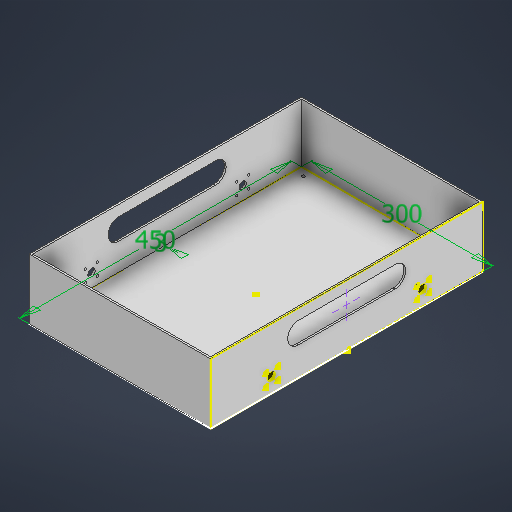
# Autodesk Inventor part: AMR_Base_Box_V2
Saved by Autodesk Inventor 2026.2 (Build 302298010, 298A)
## iProperties
Created: 2026-03-25
Part Number: AMR_Base_Box_V2
Material: Generic
Document SubType Name: Modeling
Designer: Srishanth Dhondy
Density: 1 g/cm^3
Appearance: Default
Author: Srishanth Dhondy
Autodesk Inventor part; units mm, degrees
ref_plane "YZ Plane" through (0, 0, 0) normal (1, 0, 0) x (0, 1, 0)
ref_plane "XZ Plane" through (0, 0, 0) normal (0, 1, 0) x (-1, 0, 0)
ref_plane "XY Plane" through (0, 0, 0) normal (0, 0, 1) x (1, 0, 0)
sketch "Sketch1" plane through (0, 0, 0) normal (0, 1, 0) x (-1, 0, 0)
  line L0 (-150, 225) -> (150, 225)
  line L1 (150, 225) -> (150, -225)
  line L2 (150, -225) -> (-150, -225)
  line L3 (-150, -225) -> (-150, 225)
  line L4 (-150, 225) -> (150, -225) construction
  line L5 (150, 225) -> (-150, -225) construction
  line L6 (147, -222) -> (147, 222)
  line L7 (147, 222) -> (-147, 222)
  line L8 (-147, 222) -> (-147, -222)
  line L9 (-147, -222) -> (147, -222)
  point P0 (0, 0)
  dimension "d0" = 300
  dimension "d1" = 450
  dimension "d4" = 3
  constraints: 20 end point, 4 parallel, 2 midpoint, 2 perpendicular, 1 horizontal, 3 other
  measures "d0" distance of L1.end L2.end
  measures "d1" distance of L0.end L1.end
  measures "d4" distance between parallel lines of L1 L6
extrude "Extrusion1" add sketch "Sketch1" along normal blind 3 contours L0 L1 L2 L3 | L9 L8 L7 L6
extrude "Extrusion2" add sketch "Sketch1" along normal blind 100
sketch "Sketch2" plane through (150, 0, 225) normal (1, 0, 0) x (0, 0, -1)
  line L0 (0, 0) -> (450, 0) projected
  line L1 (450, 0) -> (450, 100) projected
  line L2 (0, 100) -> (450, 100) projected
  line L3 (0, 0) -> (0, 100) projected
  line L4 (0, 25) -> (450, 25)
  circle A0 centre (100, 25) radius 14
  circle A1 centre (350, 25) radius 14
  line L5 (100, 25) -> (109.8995, 34.8995) construction
  line L6 (100, 25) -> (114, 25) construction
  line L7 (225, 100) -> (225, 0) construction
  circle A2 centre (100, 25) radius 6
  circle A3 centre (350, 25) radius 6
  point P0 (90.1005, 34.8995)
  point P1 (90.1005, 15.1005)
  point P2 (109.8995, 15.1005)
  point P3 (340.1005, 34.8995)
  point P4 (359.8995, 34.8995)
  point P5 (359.8995, 15.1005)
  point P6 (340.1005, 15.1005)
  dimension "d7" = 28
  dimension "d8" = 28
  dimension "d9" = 45
  dimension "d12" = 360
  dimension "d14" = 12
  dimension "d15" = 12
  constraints: 13 coincident, 8 end point, 4 point on line, 4 symmetric about line, 3 centre point, 2 perpendicular, 1 equal length, 1 horizontal, 1 midpoint, 8 other
  measures "d8" diameter of A1
  measures "d9" angle of L6 L5
  measures "d14" diameter of A2
  measures "d15" diameter of A3
hole "Hole1" at (150, 25, 125) at (150, 25, -125) direction (-1, 0, 0) diameter 12 end through all
hole "Hole2" at (150, 34.8995, 134.8995) at (150, 15.1005, 115.1005) at (150, 15.1005, 134.8995) at (150, 34.8995, 115.1005) at (150, 34.8995, -115.1005) at (150, 15.1005, -115.1005) at (150, 15.1005, -134.8995) at (150, 34.8995, -134.8995) direction (-1, 0, 0) diameter 3.5 end through all
sketch "Sketch3" plane through (0, 3, 0) normal (0, 1, 0) x (1, 0, 0)
  line L0 (-147, 222) -> (-147, -222) projected
  line L1 (-147, -222) -> (147, -222) projected
  line L2 (147, -222) -> (147, 222) projected
  line L3 (147, 222) -> (-147, 222) projected
  point P0 (0, 0)
sketch "Sketch4" plane through (0, 3, 0) normal (0, 1, 0) x (1, 0, 0)
  line L0 (-147, 222) -> (-147, -222) projected
  line L1 (147, -222) -> (147, 222) projected
  line L2 (150, 225) -> (-150, 225) projected
  line L3 (0, 225) -> (0, -313.1103)
  line L4 (-147, 0) -> (147, 0)
  point P0 (0, 0)
  point P1 (-202.9851, -76.8809)
  point P2 (132, 256.112)
  point P3 (-124.075, 248.076)
  point P4 (-124.075, -228.643)
  point P5 (147.6668, -220.1737)
  point P6 (132, 210)
  point P7 (-132, 210)
  point P8 (132, -210)
  point P9 (-132, -210)
  dimension "d30" = 132
  dimension "d31" = 210
  constraints: 4 end point, 3 midpoint, 3 symmetric about line, 1 vertical
  measures "d30" distance from line of point (132, 256.112) L3
  measures "d31" distance from line of point (132, 210) L4
hole "Hole3" at (132, 3, -210) at (-132, 3, -210) at (-132, 3, 210) at (132, 3, 210) direction (0, -1, 0) diameter 5 end through all
sketch "Sketch5" plane through (150, 0, 225) normal (1, 0, 0) x (0, 0, -1)
  circle A0 centre (359.8995, 34.8995) radius 1.75 projected
  circle A1 centre (359.8995, 15.1005) radius 1.75 projected
  circle A2 centre (340.1005, 15.1005) radius 1.75 projected
  circle A3 centre (340.1005, 34.8995) radius 1.75 projected
  circle A4 centre (109.8995, 34.8995) radius 1.75 projected
  circle A5 centre (90.1005, 15.1005) radius 1.75 projected
  circle A6 centre (109.8995, 15.1005) radius 1.75 projected
  circle A7 centre (90.1005, 34.8995) radius 1.75 projected
  circle A8 centre (350, 25) radius 6 projected
  circle A9 centre (100, 25) radius 6 projected
  line L0 (0, 0) -> (450, 0) projected
  line L1 (450, 0) -> (450, 100) projected
  line L2 (0, 100) -> (450, 100) projected
  line L3 (0, 0) -> (0, 100) projected
  point P0 (225, 0)
  point P1 (225, 65)
  point P2 (225, 65)
  constraints: 1 coincident
sketch "Sketch6" plane through (150, 0, 225) normal (1, 0, 0) x (0, 0, -1)
  circle A0 centre (359.8995, 34.8995) radius 1.75 projected
  circle A1 centre (359.8995, 15.1005) radius 1.75 projected
  circle A2 centre (340.1005, 15.1005) radius 1.75 projected
  circle A3 centre (340.1005, 34.8995) radius 1.75 projected
  circle A4 centre (109.8995, 34.8995) radius 1.75 projected
  circle A5 centre (90.1005, 15.1005) radius 1.75 projected
  circle A6 centre (109.8995, 15.1005) radius 1.75 projected
  circle A7 centre (90.1005, 34.8995) radius 1.75 projected
  circle A8 centre (350, 25) radius 6 projected
  circle A9 centre (100, 25) radius 6 projected
  line L0 (0, 0) -> (450, 0) projected
  line L1 (450, 0) -> (450, 100) projected
  line L2 (0, 100) -> (450, 100) projected
  line L3 (0, 0) -> (0, 100) projected
  point P0 (225, 0)
sketch "Sketch7" plane through (150, 0, 225) normal (1, 0, 0) x (0, 0, -1)
  line L0 (145, 65.0001) -> (305, 65.0001) construction
  line L1 (145, 47.5001) -> (305, 47.5001)
  line L2 (305, 82.5001) -> (145, 82.5001)
  arc A0 (145, 82.5001) -> (145, 47.5001) centre (145, 65.0001) ccw
  arc A1 (305, 47.5001) -> (305, 82.5001) centre (305, 65.0001) ccw
  point P0 (225, 0)
  point P1 (225, 65.0001)
  dimension "d42" = 80
  dimension "d43" = 35
  constraints: 8 end point, 4 point on circle, 4 tangent, 2 centre point, 1 horizontal, 1 midpoint, 1 parallel
  measures "d42" distance of point (225, 65) L0.end
  measures "d43" diameter of A1
extrude "Extrusion3" cut sketch "Sketch7" against normal through all
body "Solid1"
